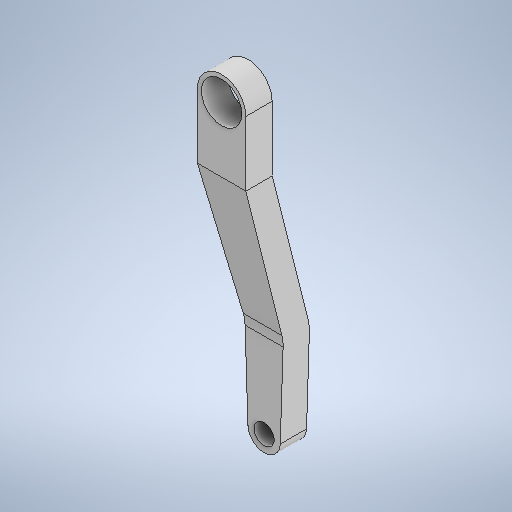
# Autodesk Inventor part: 47A
Saved by Autodesk Inventor 2025.1 (Build 291241000, 241)
## iProperties
Created: 2024-09-17
Part Number: 47A
Material: Generisch
Document SubType Name: Modeling
Designer: ffogue
Density: 1 g/cm^3
Appearance: Vorgabe
Author: ffogue
Autodesk Inventor part; units mm, degrees
ref_plane "YZ Plane" through (0, 0, 0) normal (1, 0, 0) x (0, 1, 0)
ref_plane "XZ Plane" through (0, 0, 0) normal (0, 1, 0) x (-1, 0, 0)
ref_plane "XY Plane" through (0, 0, 0) normal (0, 0, 1) x (1, 0, 0)
sketch "Sketch19" plane through (0, 0, 0) normal (1, 0, 0) x (0, 1, 0)
  line L0 (0, 0) -> (0, -22)
  line L1 (0, -22) -> (10.1375, -58.6184)
  line L2 (10.5, -61.2865) -> (10.5, -86.2865)
  line L3 (10.5, -86.2865) -> (17, -86.2865)
  line L4 (17, -86.2865) -> (17, -61.2865)
  line L5 (16.6375, -58.6184) -> (6.5, -22)
  line L6 (6.5, -22) -> (6.5, 0)
  line L7 (6.5, 0) -> (0, 0)
  arc A0 (10.5, -61.2865) -> (10.1375, -58.6184) centre (0.5, -61.2865) ccw
  arc A1 (17, -61.2865) -> (16.6375, -58.6184) centre (7, -61.2865) ccw
  point P0 (16.909, -59.9402)
  dimension "d79" = 10
  dimension "d80" = 10
  dimension "d82" = 6.5
  dimension "d83" = 10.5
  dimension "d84" = 25
  dimension "d85" = 22
  dimension "d86" = 37.9402
  constraints: 16 end point, 5 point on circle, 4 tangent, 3 parallel, 3 perpendicular, 2 centre point, 2 horizontal alignment, 1 vertical
  measures "d79" radius of A0
  measures "d80" radius of A1
  measures "d82" distance of L6.end L0.start
  measures "d83" distance between parallel lines of L0 L2
  measures "d84" distance of L3.end L4.end
  measures "d85" distance of L5.end L6.end
  measures "d86" vertical distance of point (16.909, -59.94) L5.end
extrude "Extrusion7" add sketch "Sketch19" along normal blind 12
sketch "Sketch20" plane through (0, 6.5, 0) normal (0, 1, 0) x (1, 0, 0)
  circle A0 centre (6, 6) radius 6
  line L0 (0, 0) -> (12, 0) projected
  line L1 (0, 0) -> (12, 0) projected
  line L2 (0, 0) -> (0, 6)
  line L3 (0, 0) -> (0, 22) projected
  line L4 (12, 0) -> (12, 6)
  point P0 (6, 0)
  point P1 (6, 0)
  dimension "d89" = 12
  constraints: 4 end point, 3 point on circle, 2 midpoint, 1 centre point, 1 point on line, 1 tangent, 1 vertical alignment
  measures "d89" diameter of A0
extrude "Extrusion8" cut sketch "Sketch20" against normal blind 12 contours L4 L0 A0 | A0 L0 L2
sketch "Sketch21" plane through (0, 17, -61.2865) normal (0, 1, 0) x (1, 0, 0)
  circle A0 centre (6, 21) radius 4
  line L0 (0, 25) -> (12, 25) projected
  arc A1 (0, -55.2865) -> (12, -55.2865) centre (6, -55.2865) ccw projected
  line L1 (12, -39.2865) -> (12, -55.2865) projected
  line L2 (0, -39.2865) -> (12, -39.2865) projected
  line L3 (0, -39.2865) -> (0, -55.2865) projected
  line L4 (0, -39.2865) -> (2.0022, 21.1325)
  line L5 (12, -39.2865) -> (12, -2.6681) projected
  line L6 (12, -39.2865) -> (9.9978, 21.1325)
  line L7 (0, 25) -> (0, 0) projected
  line L8 (0, -39.2865) -> (0, 25)
  line L9 (0, 25) -> (6, 25)
  line L10 (6, 25) -> (12, 25)
  line L11 (12, 0) -> (12, 25) projected
  line L12 (12, 25) -> (12, -39.2865)
  point P0 (0, -61.2865)
  point P1 (12, 0)
  dimension "d93" = 8
  constraints: 12 end point, 4 tangent, 3 collinear, 3 point on circle, 2 midpoint, 1 centre point, 1 perpendicular, 1 vertical alignment
  measures "d93" diameter of A0
extrude "Extrusion9" cut sketch "Sketch21" against normal up to surface (17 mm away) contours A0 L0 L11 L12 L5 L6 | L4 L8 L7 L0 A0
sketch "Sketch22" plane through (6, 6.5, -6) normal (0, 1, 0) x (1, 0, 0)
  arc A0 (-6, 0) -> (6, 0) centre (0, 0) ccw projected
  point P0 (-6, -6)
  constraints: 1 coincident
hole "Hole1" at (6, 6.5, -6) direction (0, -1, 0) diameter 10 end through all
sketch "Sketch23" plane through (6, 17, -82.2865) normal (0, 1, 0) x (1, 0, 0)
  arc A0 (3.9978, 0.1325) -> (-3.9978, 0.1325) centre (0, 0) ccw projected
  point P0 (-6, -82.2865)
  constraints: 1 coincident
hole "Hole2" at (6, 17, -82.2865) direction (0, -1, 0) diameter 5 end through all
fillet "Fillet1" radius 10 1 edges at (6, 6.5, -22)
body "Solid2"
